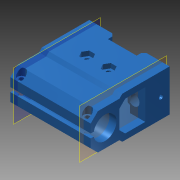
# Autodesk Inventor part: XCarriage
Saved by Autodesk Inventor 2015 (Build 190159000, 159)
## iProperties
Created: 2014-08-15
Part Number: XCarriage
Material: ABS Plastic
Document SubType Name: Modeling
Designer: t_clevj
Density: 1.06 g/cm^3
Appearance: Cyan
Author: t_clevj
Autodesk Inventor part; units mm, degrees
ref_plane "YZ Plane" through (0, 0, 0) normal (1, 0, 0) x (0, 1, 0)
ref_plane "XZ Plane" through (0, 0, 0) normal (0, 1, 0) x (-1, 0, 0)
ref_plane "XY Plane" through (0, 0, 0) normal (0, 0, 1) x (1, 0, 0)
sketch "Sketch1" plane through (0, 0, 0) normal (1, 0, 0) x (0, 1, 0)
  arc A0 (-7.8581, -1.5) -> (-7.8581, 1.5) centre (0, 0) ccw
  line L0 (-10, 1.5) -> (-10, 12.5)
  line L1 (-10, 12.5) -> (40, 12.5)
  line L2 (-10, -1.5) -> (-10, -12.5)
  line L3 (-10, -12.5) -> (40, -12.5)
  line L4 (-10, 1.5) -> (-7.8581, 1.5)
  line L5 (-10, -1.5) -> (-7.8581, -1.5)
  line L6 (40, 12.5) -> (40, -12.5)
  dimension "d0" = 16
  dimension "d1" = 1.5
  dimension "d2" = 1.5
  dimension "d3" = 10
  dimension "d4" = 12.5
  dimension "d5" = 12.5
  dimension "d6" = 50
  constraints: 14 end point, 3 vertical, 2 horizontal, 2 point on circle, 2 vertical alignment, 1 centre point, 1 coincident, 1 parallel, 1 perpendicular
  measures "d0" diameter of A0
  measures "d1" vertical distance of point (0, 0) L2.start
  measures "d2" vertical distance of point (0, 0) L0.start
  measures "d3" distance from line of point (0, 0) L0
  measures "d4" distance from line of point (0, 0) L1
  measures "d5" distance from line of L3 point (0, 0)
  measures "d6" distance of L0.end L1.end
extrude "MainBlock" add sketch "Sketch1" along normal blind 56
chamfer "BearingHolderChamfer" distance 5 angle 45 2 edges at (28, -10, 12.5) (28, -10, -12.5)
sketch "Sketch2" plane through (0, 40, 12.5) normal (0, 0, 1) x (1, 0, 0)
  line L0 (56, -50) -> (56, -45) projected
  line L1 (56, -45) -> (0, -45) projected
  line L2 (0, -45) -> (0, -50) projected
  line L3 (0, -50) -> (56, -50) projected
  point P0 (0, -40)
  point P1 (5, -47.25)
  point P2 (51, -47.25)
  dimension "d17" = 2.75
  dimension "d18" = 5
  dimension "d19" = 5
  constraints: 1 horizontal alignment
  measures "d17" distance from line of L3 point (51, -47.25)
  measures "d18" distance from line of L0 point (51, -47.25)
  measures "d19" distance from line of L2 point (5, -47.25)
hole "BearingHolderClamp" at (5, -7.25, 12.5) at (51, -7.25, 12.5) direction (0, 0, -1) diameter 3 depth 25 tip angle 118 counterbore diameter 5.5 counterbore depth 5
sketch "Sketch3" plane through (56, 40, -12.5) normal (0, 0, -1) x (-1, 0, 0)
  circle A0 centre (51, -47.25) radius 1.5 projected
  arc A1 (49.6288, -47.8581) -> (52.3712, -47.8581) centre (51, -47.25) ccw projected
  circle A2 centre (5, -47.25) radius 1.5 projected
  arc A3 (3.6288, -47.8581) -> (6.3712, -47.8581) centre (5, -47.25) ccw projected
  line L0 (8.1754, -47.25) -> (6.5877, -50)
  line L1 (6.5877, -50) -> (3.4123, -50)
  line L2 (3.4123, -50) -> (1.8246, -47.25)
  line L3 (1.8246, -47.25) -> (3.4123, -44.5)
  line L4 (3.4123, -44.5) -> (6.5877, -44.5)
  line L5 (6.5877, -44.5) -> (8.1754, -47.25)
  line L6 (54.1754, -47.25) -> (52.5877, -50)
  line L7 (52.5877, -50) -> (49.4123, -50)
  line L8 (49.4123, -50) -> (47.8246, -47.25)
  line L9 (47.8246, -47.25) -> (49.4123, -44.5)
  line L10 (49.4123, -44.5) -> (52.5877, -44.5)
  line L11 (52.5877, -44.5) -> (54.1754, -47.25)
  point P0 (56, -40)
  dimension "d27" = 5.5
  dimension "d28" = 5.5
  constraints: 24 end point, 2 coincident, 2 horizontal, 2 horizontal alignment, 26 other
  measures "d27" distance between parallel lines of L1 L4
  measures "d28" distance between parallel lines of L7 L10
extrude "BearingHolderNutTrap" cut sketch "Sketch3" against normal blind 5
sketch "Sketch4" plane through (0, 0, 0) normal (-1, 0, 0) x (0, 0, 1)
  arc A0 (1.5, -7.8581) -> (-1.5, -7.8581) centre (0, 0) ccw projected
  line L0 (-12.5, 40) -> (-12.5, -5) projected
  line L1 (10.5, 10) -> (-10.5, 10)
  line L2 (-10.5, 10) -> (-10.5, 28)
  line L3 (-10.5, 28) -> (10.5, 28)
  line L4 (10.5, 28) -> (10.5, 10)
  dimension "d31" = 18
  dimension "d32" = 21
  dimension "d33" = 10
  dimension "d34" = 2
  constraints: 8 end point, 2 parallel, 1 horizontal, 1 perpendicular
  measures "d31" distance of L1.end L2.end
  measures "d32" distance of L1.start L1.end
  measures "d33" distance from line of A0.centre L1
  measures "d34" distance between parallel lines of L0 L2
extrude "BeltCutoutY" cut sketch "Sketch4" against normal up to surface (56 mm away)
sketch "Sketch5" plane through (0, 40, 12.5) normal (0, 1, 0) x (1, 0, 0)
  line L0 (56, 25) -> (56, 0) projected
  line L1 (0, 25) -> (56, 25) projected
  line L2 (18, 2) -> (38, 2)
  line L3 (38, 2) -> (38, 23)
  line L4 (38, 23) -> (18, 23)
  line L5 (18, 23) -> (18, 2)
  point P0 (0, 12.5)
  dimension "d37" = 21
  dimension "d38" = 20
  dimension "d39" = 2
  dimension "d40" = 18
  constraints: 8 end point, 2 parallel, 1 horizontal, 1 perpendicular
  measures "d37" distance of L4.end L2.start
  measures "d38" distance of L2.start L2.end
  measures "d39" distance between parallel lines of L1 L4
  measures "d40" distance between parallel lines of L0 L3
extrude "BeltCutoutX" cut sketch "Sketch5" against normal up to surface (12 mm away)
sketch "Sketch6" plane through (56, 40, -12.5) normal (0, 0, -1) x (-1, 0, 0)
  line L0 (56, 0) -> (56, -45) projected
  line L1 (56, 0) -> (0, 0) projected
  line L2 (0, -45) -> (0, 0) projected
  line L3 (0, -28) -> (56, -28)
  point P0 (56, -40)
  dimension "d43" = 28
  constraints: 2 end point, 2 point on line, 1 perpendicular
  measures "d43" distance between parallel lines of L1 L3
extrude "BoltPadUpper" add sketch "Sketch6" along normal blind 2
sketch "Sketch7" plane through (0, 40, 12.5) normal (0, 0, 1) x (1, 0, 0)
  line L0 (56, 0) -> (56, -45) projected
  line L1 (0, 0) -> (56, 0) projected
  line L2 (0, -45) -> (0, 0) projected
  line L3 (0, -28) -> (0, 0) projected
  line L4 (0, -28) -> (56, -28)
  line L5 (56, 0) -> (56, -28) projected
  point P0 (0, -40)
  dimension "d46" = 28
  constraints: 2 end point, 2 point on line, 1 perpendicular
  measures "d46" distance between parallel lines of L1 L4
extrude "BoltPadLower" add sketch "Sketch7" along normal blind 2
chamfer "BoltPadChamfer" distance 2 angle 45 2 edges at (28, 12, 12.5) (28, 12, -12.5)
sketch "Sketch8" plane through (56, 40, -14.5) normal (0, 0, -1) x (-1, 0, 0)
  line L0 (56, 0) -> (0, 0) projected
  line L1 (0, 0) -> (0, -28) projected
  point P0 (56, -40)
  point P1 (20.5, -17)
  point P2 (35.5, -17)
  dimension "d54" = 17
  dimension "d116" = 15
  dimension "d117" = 20.5
  constraints: 1 horizontal alignment
  measures "d54" distance from line of L0 point (35.5, -17)
  measures "d116" distance of point (35.5, -17) point (20.5, -17)
  measures "d117" distance from line of L1 point (20.5, -17)
hole "BearingBoltHoles" at (35.5, 23, -14.5) at (20.5, 23, -14.5) direction (0, 0, 1) diameter 4 end up to face face through (18.6667, 21.3333, 14.5) facing (0, 0, 1) counterbore diameter 7 counterbore depth 1.5
chamfer "BearingCutoutYChamfer" distance 4 angle 45 2 edges at (28, 10, 10.5) (28, 10, -10.5)
sketch "Sketch9" plane through (38, 40, 10.5) normal (0, 0, -1) x (-1, 0, 0)
  line L0 (38, -12) -> (20, -12) projected
  line L1 (20, 0) -> (20, -12) projected
  line L2 (0, 0) -> (0, -12) projected
  line L3 (0, -12) -> (-18, -12) projected
  circle A0 centre (17.5, -17) radius 2 projected
  circle A1 centre (2.5, -17) radius 2 projected
  arc A2 (0, -6.2879) -> (-7.298, -12) centre (2.5, -17) ccw
  arc A3 (27.298, -12) -> (20, -6.2879) centre (17.5, -17) ccw
  point P0 (38, -40)
  dimension "d67" = 11
  dimension "d68" = 11
  constraints: 4 point on circle, 4 point on line, 2 centre point, 2 coincident
  measures "d67" radius of A3
  measures "d68" radius of A2
extrude "BearingClearanceCut" cut sketch "Sketch9" along normal up to surface (21 mm away) contours L0 L1 A3 | L2 L3 A2
sketch "Sketch10" plane through (0, 40, 14.5) normal (0, 0, 1) x (1, 0, 0)
  circle A0 centre (35.5, -17) radius 2 projected
  circle A1 centre (20.5, -17) radius 2 projected
  line L0 (24.5415, -17) -> (22.5207, -20.5)
  line L1 (22.5207, -20.5) -> (18.4793, -20.5)
  line L2 (18.4793, -20.5) -> (16.4585, -17)
  line L3 (16.4585, -17) -> (18.4793, -13.5)
  line L4 (18.4793, -13.5) -> (22.5207, -13.5)
  line L5 (22.5207, -13.5) -> (24.5415, -17)
  line L6 (39.5415, -17) -> (37.5207, -20.5)
  line L7 (37.5207, -20.5) -> (33.4793, -20.5)
  line L8 (33.4793, -20.5) -> (31.4585, -17)
  line L9 (31.4585, -17) -> (33.4793, -13.5)
  line L10 (33.4793, -13.5) -> (37.5207, -13.5)
  line L11 (37.5207, -13.5) -> (39.5415, -17)
  point P0 (0, -40)
  dimension "d71" = 7
  constraints: 24 end point, 2 coincident, 2 horizontal, 1 collinear, 26 other
  measures "d71" distance between parallel lines of L1 L4
extrude "BearingNutTrap" cut sketch "Sketch10" against normal blind 3.2
sketch "Sketch11" plane through (56, 40, -14.5) normal (0, 0, -1) x (-1, 0, 0)
  line L0 (56, 0) -> (0, 0) projected
  line L1 (0, 5) -> (16, 5)
  line L2 (56, 5) -> (40, 5)
  line L3 (56, 5) -> (56, 0)
  line L4 (0, 0) -> (0, 5)
  line L5 (18, 0) -> (18, 0)
  line L6 (38, 0) -> (38, 0)
  line L7 (18, 0) -> (18, 3)
  line L8 (18, 0) -> (18, -6.2879) projected
  line L9 (38, 0) -> (38, 3)
  line L10 (40, 5) -> (38, 3)
  line L11 (16, 5) -> (18, 3)
  point P0 (56, -40)
  dimension "d74" = 16
  dimension "d75" = 16
  dimension "d80" = 5
  dimension "d93" = 3
  constraints: 20 end point, 2 horizontal, 2 perpendicular, 2 vertical, 1 collinear, 1 horizontal alignment, 1 parallel, 1 point on line
  measures "d74" distance of L1.start L1.end
  measures "d75" distance of L2.start L2.end
  measures "d80" distance of L2.start L0.start
  measures "d93" distance of L5.end L7.end
extrude "XRodHolderPad" add sketch "Sketch11" against normal up to surface (29 mm away)
sketch "Sketch15" plane through (0, 45, -14.5) normal (0, 1, 0) x (1, 0, 0)
  line L0 (0, -29) -> (16, -29) projected
  line L1 (0, 0) -> (0, -29) projected
  line L2 (40, -29) -> (56, -29) projected
  line L3 (56, 0) -> (56, -29) projected
  line L4 (40, 0) -> (56, 0) projected
  line L5 (40, 0) -> (40, -29) projected
  circle A0 centre (8, -13.5) radius 4
  circle A1 centre (48, -13.5) radius 4
  point P0 (0, -14.5)
  dimension "d94" = 8
  dimension "d95" = 8
  dimension "d96" = 8
  dimension "d97" = 8
  dimension "d98" = 15.5
  dimension "d99" = 15.5
  constraints: 2 centre point
  measures "d94" diameter of A0
  measures "d95" diameter of A1
  measures "d96" distance from line of L1 A0.centre
  measures "d97" distance from line of L3 A1.centre
  measures "d98" distance from line of L0 A0.centre
  measures "d99" distance from line of L2 A1.centre
extrude "XRodHole" cut sketch "Sketch15" against normal up to surface (17 mm away) contours A0 | A1
sketch "Sketch16" plane through (0, 0, 0) normal (-1, 0, 0) x (0, 0, 1)
  line L0 (14.5, 12) -> (14.5, 45) projected
  line L1 (-14.5, 45) -> (14.5, 45) projected
  circle A0 centre (-1, 39) radius 1.5
  dimension "d102" = 3
  dimension "d103" = 6
  dimension "d104" = 15.5
  constraints: 1 centre point
  measures "d102" diameter of A0
  measures "d103" distance from line of L1 A0.centre
  measures "d104" distance from line of L0 A0.centre
extrude "XRodSetScrewLeft" cut sketch "Sketch16" against normal up to next
sketch "Sketch17" plane through (56, 0, 0) normal (1, 0, 0) x (0, 0, -1)
  line L0 (14.5, 45) -> (-14.5, 45) projected
  line L1 (-14.5, 12) -> (-14.5, 45) projected
  circle A0 centre (1, 39) radius 1.5
  dimension "d107" = 3
  dimension "d108" = 6
  dimension "d109" = 15.5
  constraints: 1 centre point
  measures "d107" diameter of A0
  measures "d108" distance from line of L0 A0.centre
  measures "d109" distance from line of L1 A0.centre
extrude "XRodSetScrewRight" cut sketch "Sketch17" against normal up to next
ref_plane "Work Plane1" through (5, 0, 0) normal (-1, 0, 0) x (0, 0, 1)
sketch "Sketch18" plane through (5, 0, 0) normal (-1, 0, 0) x (0, 0, 1)
  circle A0 centre (-1, 39) radius 1.5 projected
  line L0 (-1, 35.8246) -> (-3.75, 37.4123)
  line L1 (-3.75, 37.4123) -> (-3.75, 40.5877)
  line L2 (-3.75, 40.5877) -> (-1, 42.1754)
  line L3 (-1, 42.1754) -> (1.75, 40.5877)
  line L4 (1.75, 40.5877) -> (1.75, 37.4123)
  line L5 (1.75, 37.4123) -> (-1, 35.8246)
  point P0 (0, 0)
  dimension "d113" = 5.5
  constraints: 12 end point, 1 coincident, 1 vertical, 14 other
  measures "d113" distance between parallel lines of L4 L1
extrude "XRodSetScrewNutTrapLeft" cut sketch "Sketch18" along normal blind 3.5
ref_plane "Work Plane2" through (51, 0, 0) normal (1, 0, 0) x (0, 0, -1)
sketch "Sketch19" plane through (51, 0, 0) normal (1, 0, 0) x (0, 0, -1)
  spline S0 degree 2 poles (-0.5, 39) (-0.5, 41.5981) (1.75, 40.299) (4, 39) (1.75, 37.701) (-0.5, 36.4019) (-0.5, 39) knots 0 0 0 0.333333 0.333333 0.666667 0.666667 1 1 1 weights 1 0.5 1 0.5 1 0.5 1 projected
  circle A0 centre (1, 39) radius 1.5 projected
  line L0 (1, 42.1754) -> (3.75, 40.5877)
  line L1 (3.75, 40.5877) -> (3.75, 37.4123)
  line L2 (3.75, 37.4123) -> (1, 35.8246)
  line L3 (1, 35.8246) -> (-1.75, 37.4123)
  line L4 (-1.75, 37.4123) -> (-1.75, 40.5877)
  line L5 (-1.75, 40.5877) -> (1, 42.1754)
  point P0 (0, 0)
  dimension "d119" = 5.5
  constraints: 12 end point, 1 coincident, 1 horizontal alignment, 1 vertical, 14 other
  measures "d119" distance between parallel lines of L4 L1
extrude "XRodSetScrewNutTrapRight" cut sketch "Sketch19" along normal blind 3.5
body "Solid1"
